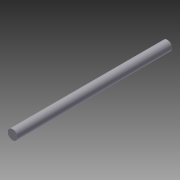
# Autodesk Inventor part: AWI-12
Saved by Autodesk Inventor 2011 (Build 150239000, 239)
## iProperties
Category: Plastic Bearings
Created: 2007-11-11
Part Number: AWI-12
Material: Aluminum-6061
Catalog Web Link: http://www.igus.com/drylins.asp
Description: Drylin S Aluminum Shaft
Vendor: igus
Document SubType Name: Modeling
Mass: 235.431 g
Surface Area: 188.115 cm^2
Volume: 86.875 cm^3
Density: 2.71 g/cm^3
Project: FIRST
Title: Drylin S Aluminum Shaft
Author: Autodesk, Inc.
Autodesk Inventor part; units mm, degrees
ref_plane "YZ Plane" through (0, 0, 0) normal (1, 0, 0) x (0, 1, 0)
ref_plane "XZ Plane" through (0, 0, 0) normal (0, 1, 0) x (-1, 0, 0)
ref_plane "XY Plane" through (0, 0, 0) normal (0, 0, 1) x (1, 0, 0)
sketch "Sketch1" plane through (0, 0, 0) normal (0, 0, 1) x (1, 0, 0)
  circle A0 centre (0, 0) radius 9.525
  dimension "d0" = 19.05
  dimension "d0" = 19.05
  constraints: 1 centre point, 1 coincident
  measures "d0" diameter of A0
extrude "Extrusion1" add sketch "Sketch1" along normal blind 304.8
body "Solid1"
